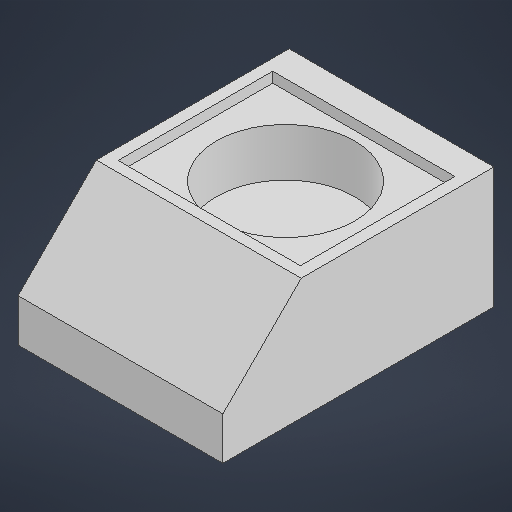
# Autodesk Inventor part: Spin Coater
Saved by Autodesk Inventor 2025.1 (Build 291241000, 241)
## iProperties
Created: 2025-02-09
Part Number: Spin Coater
Material: Generic
Document SubType Name: Modeling
Designer: jerem
Density: 1 g/cm^3
Appearance: Default
Author: jerem
Autodesk Inventor part; units mm, degrees
ref_plane "YZ Plane" through (0, 0, 0) normal (1, 0, 0) x (0, 1, 0)
ref_plane "XZ Plane" through (0, 0, 0) normal (0, 1, 0) x (-1, 0, 0)
ref_plane "XY Plane" through (0, 0, 0) normal (0, 0, 1) x (1, 0, 0)
sketch "Sketch1" plane through (0, 0, 0) normal (0, 1, 0) x (-1, 0, 0)
  line L0 (-85, 112.5) -> (85, 112.5)
  line L1 (85, 112.5) -> (85, -112.5)
  line L2 (85, -112.5) -> (-85, -112.5)
  line L3 (-85, -112.5) -> (-85, 112.5)
  line L4 (-85, 112.5) -> (85, -112.5) construction
  line L5 (85, 112.5) -> (-85, -112.5) construction
  circle A0 centre (69.3, 81.8) radius 2.5
  circle A1 centre (69.3, -81.8) radius 2.5
  circle A2 centre (-69.3, -81.8) radius 2.5
  circle A3 centre (-69.3, 81.8) radius 2.5
  line L6 (69.3, 81.8) -> (-69.3, 81.8) construction
  line L7 (69.3, 81.8) -> (69.3, -81.8) construction
  line L8 (69.3, -81.8) -> (-69.3, -81.8) construction
  line L9 (69.3, 0) -> (0, 0) construction
  line L10 (0, 81.8) -> (0, 0) construction
  dimension "d2" = 170
  dimension "d3" = 225
  dimension "d9" = 163.6
  dimension "d10" = 5
  dimension "d11" = 138.6
  constraints: 22 end point, 4 centre point, 4 horizontal, 4 midpoint, 3 equal radius, 3 parallel, 3 perpendicular
  measures "d2" distance of L1.end L2.end
  measures "d3" distance of L0.end L1.end
  measures "d9" distance of L6.start L7.end
  measures "d10" diameter of A0
  measures "d11" distance of L6.start L6.end
extrude "Extrusion1" add sketch "Sketch1" along normal blind 100.5 contours L0 L1 L2 L3 | A0 | A1 | A2 | A3
extrude "Extrusion2" cut sketch "Sketch1" along normal blind 10 contours A0 | A1 | A2 | A3
chamfer "Chamfer1" distance 65 angle 45 1 edges at (0, 100.5, 112.5)
sketch "Sketch2" plane through (0, 100.5, 0) normal (0, 1, 0) x (1, 0, 0)
  line L0 (75.65, -38.8) -> (-75.65, -38.8)
  line L1 (-75.65, -38.8) -> (-75.65, 89.5)
  line L2 (-75.65, 89.5) -> (75.65, 89.5)
  line L3 (75.65, 89.5) -> (75.65, -38.8)
  line L4 (75.65, -38.8) -> (-75.65, 89.5) construction
  line L5 (-75.65, -38.8) -> (75.65, 89.5) construction
  line L6 (85, -47.5) -> (-85, -47.5) projected
  line L7 (85, -47.5) -> (85, 112.5) projected
  line L8 (85, 112.5) -> (-85, 112.5) projected
  line L9 (-85, 112.5) -> (-85, -47.5) projected
  line L10 (0, 89.5) -> (0, 112.5) construction
  circle A0 centre (0, 24.5) radius 57.5
  line L11 (0, 24.5) -> (0, 82) construction
  line L12 (0, 82) -> (0, 89.5) construction
  point P0 (0, 0)
  dimension "d21" = 115
  dimension "d18" = 151.3
  dimension "d19" = 128.3
  dimension "d20" = 23
  dimension "d22" = 7.5
  constraints: 18 end point, 3 vertical, 2 midpoint, 2 parallel, 1 horizontal, 1 perpendicular, 1 vertical alignment, 2 other
  measures "d18" distance of L0.start L0.end
  measures "d19" distance of L0.end L1.end
  measures "d20" distance of L10.start L10.end
  measures "d22" distance of L10.start L11.end
extrude "Extrusion3" cut sketch "Sketch2" against normal blind 8.6 contours L0 L1 L2 L3 | A0
extrude "Extrusion4" cut sketch "Sketch2" against normal blind 40 from surface at -8.6 contours A0
body "Solid1"
